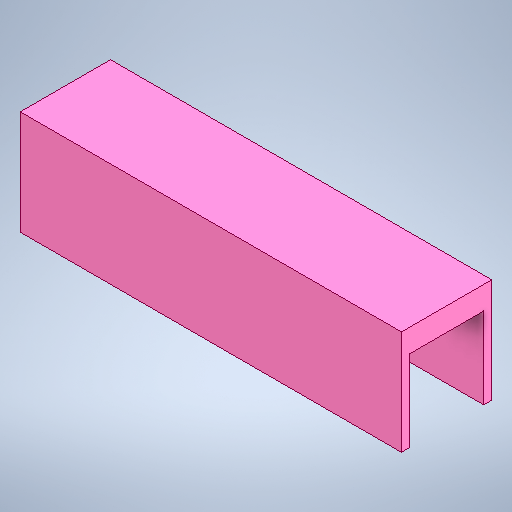
# Autodesk Inventor part: PipetteStand
Saved by Autodesk Inventor 2025.1 (Build 291241000, 241)
## iProperties
Created: 2024-11-06
Part Number: PipetteStand
Material: Generic
Document SubType Name: Modeling
Designer: 13156
Density: 1 g/cm^3
Appearance: Default
Author: 13156
Autodesk Inventor part; units mm, degrees
ref_plane "YZ Plane" through (0, 0, 0) normal (1, 0, 0) x (0, 1, 0)
ref_plane "XZ Plane" through (0, 0, 0) normal (0, 1, 0) x (-1, 0, 0)
ref_plane "XY Plane" through (0, 0, 0) normal (0, 0, 1) x (1, 0, 0)
sketch "Sketch2" plane through (0, 0, 0) normal (1, 0, 0) x (0, 1, 0)
  line L0 (26, 22.5) -> (-26, 22.5)
  line L1 (-26, 22.5) -> (-26, -22.5)
  line L2 (-26, -22.5) -> (26, -22.5)
  line L3 (26, -22.5) -> (26, 22.5)
  point P0 (0, 0)
  point P1 (-26, 0)
  point P2 (26, 0)
  dimension "d0" = 45
  dimension "d1" = 52
  dimension "d2" = 26
  dimension "d3" = 22.5
  constraints: 8 end point, 2 midpoint, 2 parallel, 1 horizontal, 1 perpendicular
  measures "d0" distance between parallel lines of L2 L0
  measures "d1" distance from line of point (-26, 0) L3
  measures "d2" distance of point (0, 0) point (26, 0)
  measures "d3" distance from line of point (0, 0) L2
extrude "Extrusion1" add sketch "Sketch2" along normal blind 125.1
sketch "Sketch3" plane through (0, -26, -22.5) normal (0, -1, 0) x (1, 0, 0)
  line L0 (125.1, 45) -> (125.1, 0) projected
  line L1 (125.1, 41) -> (5, 41)
  line L2 (5, 41) -> (5, 4)
  line L3 (5, 4) -> (125.1, 4)
  line L4 (125.1, 4) -> (125.1, 41)
  line L5 (0, 45) -> (0, 0) projected
  line L6 (0, 0) -> (125.1, 0) projected
  line L7 (0, 45) -> (125.1, 45) projected
  point P0 (0, 22.5)
  point P1 (125.1, 4)
  dimension "d6" = 5
  dimension "d7" = 37
  dimension "d8" = 4
  dimension "d45" = 4
  constraints: 8 end point, 2 parallel, 1 horizontal, 1 perpendicular, 1 point on line
  measures "d6" distance between parallel lines of L5 L2
  measures "d7" distance between parallel lines of L3 L1
  measures "d8" distance between parallel lines of L6 L3
  measures "d45" distance between parallel lines of L7 L1
extrude "Extrusion2" cut sketch "Sketch3" against normal blind 40.5 contours L0 L3 L2 L1
sketch "Sketch4" plane through (0, 0, 0) normal (-1, 0, 0) x (0, 0, 1)
  line L0 (22.5, -26) -> (18.5, -26) projected
  line L1 (-22.5, 26) -> (22.5, 26) projected
  line L2 (22.5, -26) -> (-22.5, -26)
  line L3 (-22.5, -26) -> (-22.5, 26)
  line L4 (-22.5, 26) -> (22.5, 26)
  line L5 (22.5, 26) -> (22.5, -26)
  line L6 (17.5, -26) -> (-17.5, -26)
  line L7 (-17.5, -26) -> (-17.5, 21)
  line L8 (-17.5, 21) -> (17.5, 21)
  line L9 (17.5, 21) -> (17.5, -26)
  point P0 (0, 0)
  point P1 (-17.5, -26)
  point P2 (22.5, 26)
  dimension "d11" = 5
  dimension "d12" = 5
  dimension "d13" = 5
  constraints: 16 end point, 4 parallel, 2 horizontal, 2 perpendicular, 1 point on line
  measures "d11" distance between parallel lines of L5 L9
  measures "d12" distance between parallel lines of L3 L7
  measures "d13" distance between parallel lines of L1 L8
extrude "Extrusion3" add sketch "Sketch4" along normal blind 120
sketch "Sketch5" plane through (0, 0, 0) normal (-1, 0, 0) x (0, 0, 1)
  line L0 (17.5, -26) -> (-17.5, -26) projected
  line L1 (11, -26) -> (-11, -26)
  line L2 (-11, -26) -> (-11, 9.5)
  line L3 (-11, 9.5) -> (11, 9.5)
  line L4 (11, 9.5) -> (11, -26)
  line L5 (17.5, 21) -> (17.5, -26) projected
  line L6 (-17.5, -26) -> (-17.5, 21) projected
  line L7 (-17.5, 21) -> (17.5, 21) projected
  point P0 (0, 0)
  point P1 (-11, -26)
  dimension "d16" = 6.5
  dimension "d17" = 6.5
  dimension "d18" = 11.5
  constraints: 8 end point, 2 parallel, 1 horizontal, 1 perpendicular, 1 point on line
  measures "d16" distance between parallel lines of L5 L4
  measures "d17" distance between parallel lines of L6 L2
  measures "d18" distance between parallel lines of L7 L3
extrude "Extrusion4" cut sketch "Sketch5" against normal blind 5 contours L0 L2 L3 L4
sketch "Sketch7" plane through (125.1, 0, 0) normal (1, 0, 0) x (0, 0, -1)
  line L0 (22.5, 26) -> (-22.5, 26) projected
  line L1 (22.5, -26) -> (22.5, 26) projected
  line L2 (-22.5, 26) -> (22.5, 26)
  line L3 (22.5, 26) -> (22.5, -26)
  line L4 (22.5, -26) -> (-22.5, -26)
  line L5 (-22.5, -26) -> (-22.5, 26)
  point P0 (0, 0)
  constraints: 8 end point, 2 parallel, 1 horizontal, 1 perpendicular
extrude "Extrusion6" cut sketch "Sketch7" against normal blind 55
sketch "Sketch12" plane through (0, 0, 0) normal (1, 0, 0) x (0, 0, -1)
  line L0 (-18.5, 14.5) -> (18.5, 14.5)
  line L1 (18.5, 14.5) -> (18.5, -26)
  line L2 (18.5, -26) -> (-18.5, -26)
  line L3 (-18.5, -26) -> (-18.5, 14.5)
  point P0 (0, 0)
  constraints: 8 end point, 2 parallel, 1 horizontal, 1 perpendicular
extrude "Extrusion11" cut sketch "Sketch12" against normal blind 115
sketch "Sketch13" plane through (-115, 0, 0) normal (1, 0, 0) x (0, 0, -1)
  circle A0 centre (0, 6.5) radius 1.95
  circle A1 centre (0, -18) radius 1.95
  line L0 (-18.5, 14.5) -> (18.5, 14.5) projected
  line L1 (18.5, -26) -> (-18.5, -26) projected
  point P0 (0, 0)
  dimension "d49" = 3.9
  dimension "d50" = 8
  dimension "d51" = 18.5
  dimension "d52" = 8
  dimension "d53" = 24.5
  constraints: 2 centre point, 1 equal radius
  measures "d49" diameter of A0
  measures "d50" distance from line of L0 A0.centre
  measures "d51" horizontal distance of L1.start A1.centre
  measures "d52" distance from line of L1 A1.centre
  measures "d53" distance of A1.centre A0.centre
extrude "Extrusion12" cut sketch "Sketch13" against normal blind 5
body "Solid1"
